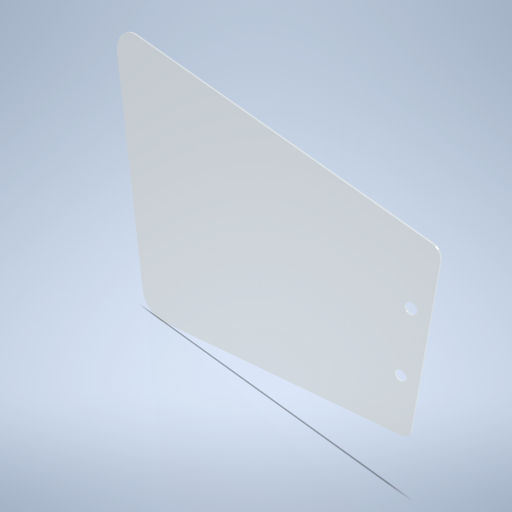
# Autodesk Inventor part: propeller_extensions
Saved by Autodesk Inventor 2024.2 (Build 282272000, 272)
## iProperties
Created: 2024-05-13
Part Number: propeller_extensions
Material: Glas
Document SubType Name: Sheet Metal
Designer: Fabri
Density: 2.18 g/cm^3
Sheet Metal Rule: Standard_mm
Appearance: Klar
Author: Fabri
Autodesk Inventor part; units mm, degrees
ref_plane "YZ Plane" through (0, 0, 0) normal (1, 0, 0) x (0, 1, 0)
ref_plane "XZ Plane" through (0, 0, 0) normal (0, 1, 0) x (-1, 0, 0)
ref_plane "XY Plane" through (0, 0, 0) normal (0, 0, 1) x (1, 0, 0)
sketch "Skizze1" plane through (0, 0, 0) normal (0, 1, 0) x (-1, 0, 0)
  line L0 (0, 25) -> (0, -25)
  line L1 (0, 25) -> (95, 45)
  line L2 (95, 45) -> (95, -45)
  line L3 (95, -45) -> (0, -25)
  point P0 (0, 0)
  point P1 (0, 0)
  dimension "d0" = 90
  dimension "d1" = 95
  dimension "d2" = 50
  measures "d0" distance of L1.end L2.end
  measures "d1" distance between parallel lines of L0 L2
  measures "d2" distance of L0.start L0.end
extrude "Grobblech1" add sketch "Skizze1" along normal mid plane 0.5
sketch "Skizze3" plane through (0, 0.25, 0) normal (0, 1, 0) x (1, 0, 0)
  line L0 (0, 25) -> (0, -25) projected
  point P0 (0, 0)
  point P1 (-4.5, -9)
  point P2 (-4.5, 9)
  dimension "d16" = 16
  dimension "d17" = 16
  dimension "d18" = 4.5
  dimension "d19" = 4.5
  measures "d16" vertical distance of L0.end point (-4.5, -9)
  measures "d17" vertical distance of L0.start point (-4.5, 9)
  measures "d18" distance from line of L0 point (-4.5, 9)
  measures "d19" distance from line of L0 point (-4.5, -9)
hole "Bohrung2" at (-4.5, 0.25, 9) at (-4.5, 0.25, -9) direction (0, -1, 0) diameter 3 end through all
fillet "Rundung1" radius 7 2 edges at (-95, 0, -45) (-95, 0, 45)
fillet "Rundung2" radius 3 2 edges at (0, 0, -25) (0, 0, 25)
equation "\"d3\" = Stärke"
equation "\"Biegeradius\" = Stärke"
equation "\"BreiteBiegungsfreistellung\" = Stärke"
equation "\"TiefeBiegungsfreistellung\" = 0.5 * Stärke"
equation "\"GrößeEckenfreistellung\" = 4 * Stärke"
equation "\"MinimalRest\" = 2 * Stärke"
equation "\"Übergangsradius\" = Biegeradius"
equation "\"JacobiRadiusGröße\" = Biegeradius"
equation "\"Abstandsgröße\" = Stärke"
equation "\"Stärke\" = 0.5"
